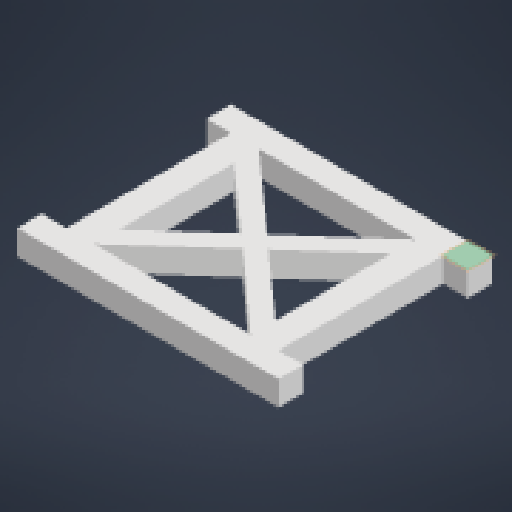
# Autodesk Inventor part: CrossReinforcement
Saved by Autodesk Inventor 2027 (Build 310192000, 192)
## iProperties
Created: 2026-04-15
Part Number: CrossReinforcement
Material: Generic
Document SubType Name: Modeling
Designer: Tueha
Density: 1 g/cm^3
Appearance: Default
Author: Tueha
Autodesk Inventor part; units mm, degrees
ref_plane "YZ Plane" through (0, 0, 0) normal (1, 0, 0) x (0, 1, 0)
ref_plane "XZ Plane" through (0, 0, 0) normal (0, 1, 0) x (-1, 0, 0)
ref_plane "XY Plane" through (0, 0, 0) normal (0, 0, 1) x (1, 0, 0)
ref_plane "Work Plane1" through (30.4614, 59.2128, -23.9588) normal (0, -1, 0) x (1, 0, 0)
sketch "Sketch1" plane through (30.4614, 59.2128, -23.9588) normal (0, -1, 0) x (1, 0, 0)
  line L0 (0, 0) -> (0, -6) projected
  line L1 (0, 0) -> (-6, 0) projected
  line L2 (-6, -6) -> (-6, 0) projected
  line L3 (0, -6) -> (-6, -6) projected
  line L4 (0, 46) -> (0, 40) projected
  line L5 (0, 46) -> (-6, 46) projected
  line L6 (-6, 40) -> (-6, 46) projected
  line L7 (0, 40) -> (-6, 40) projected
  line L8 (-57.6, 0) -> (-57.6, -6) projected
  line L9 (-57.6, 0) -> (-63.6, 0) projected
  line L10 (-63.6, -6) -> (-63.6, 0) projected
  line L11 (-57.6, -6) -> (-63.6, -6) projected
  line L12 (-57.6, 46) -> (-57.6, 40) projected
  line L13 (-57.6, 46) -> (-63.6, 46) projected
  line L14 (-63.6, 40) -> (-63.6, 46) projected
  line L15 (-57.6, 40) -> (-63.6, 40) projected
  line L16 (0, -6) -> (-6, -6)
  line L17 (-6, -6) -> (-6, 0)
  line L18 (-6, 0) -> (0, 0)
  line L19 (0, 0) -> (0, -6)
  line L20 (-63.6, -6) -> (-57.6, -6)
  line L21 (-57.6, -6) -> (-57.6, 0)
  line L22 (-57.6, 0) -> (-63.6, 0)
  line L23 (-63.6, 0) -> (-63.6, -6)
  line L24 (0, 40) -> (-6, 40)
  line L25 (-6, 40) -> (-6, 46)
  line L26 (-6, 46) -> (0, 46)
  line L27 (0, 46) -> (0, 40)
  line L28 (-63.6, 40) -> (-57.6, 40)
  line L29 (-57.6, 40) -> (-57.6, 46)
  line L30 (-57.6, 46) -> (-63.6, 46)
  line L31 (-63.6, 46) -> (-63.6, 40)
  line L32 (-6, 0) -> (-57.6, 46)
  line L33 (-6, -6) -> (-57.6, 40)
  line L34 (-57.6, 0) -> (-6, 46)
  line L35 (-6, 40) -> (-57.6, -6)
  line L36 (-6, 46) -> (-57.6, 46)
  line L37 (-6, 40) -> (-57.6, 40)
  line L38 (-57.6, -6) -> (-6, -6)
  line L39 (-6, 0) -> (-57.6, 0)
  line L40 (-50.8696, 0) -> (-50.8696, 40)
  line L41 (-12.7304, 0) -> (-12.7304, 40)
  line L42 (-57.6, 40) -> (-57.6, 0)
  line L43 (-6, 40) -> (-6, 0)
  point P0 (-30.4614, 23.9588)
  point P1 (-35.1652, 20)
  point P2 (-50.8696, 6)
  point P3 (-50.8696, 34)
  point P4 (-31.8, 23)
  point P5 (-31.8, 17)
  point P6 (-28.4348, 20)
  point P7 (-12.7304, 34)
  point P8 (-12.7304, 6)
  constraints: 56 end point, 13 parallel, 8 point on line, 5 horizontal, 5 perpendicular, 1 vertical
extrude "Extrusion1" add sketch "Sketch1" along normal blind 6 contours L0 L3 L2 L1 | L39 L41 L32 | L2 L33 L39 | L32 L41 L35 L43 | L38 L35 L39 L33 | L41 L33 L35 L32 | L37 L34 L6 | L6 L5 L4 L7 | L35 L41 L37 | L11 L10 L9 L8 | L8 L39 L35 | L35 L33 L34 L32 | L32 L34 L41 L35 | L35 L40 L34 L33 | L39 L34 L40 | L34 L37 L32 L36 | L42 L33 L40 L34 | L34 L33 L40 L32 | L32 L37 L12 | L12 L15 L14 L13 | L40 L33 L37
body "Solid1"
